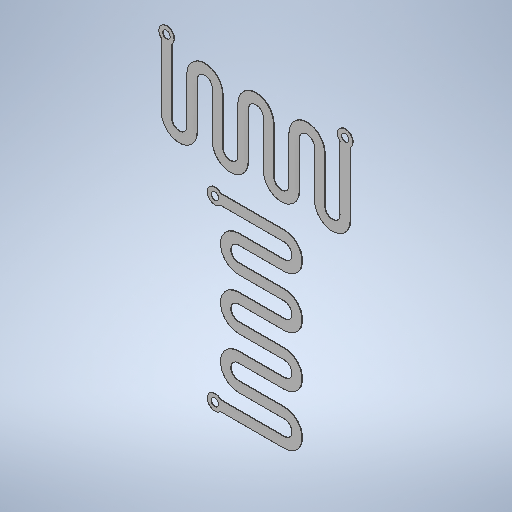
# Autodesk Inventor part: sensor_002_001
Saved by Autodesk Inventor 2025.2 (Build 292293000, 293)
## iProperties
Created: 2025-03-20
Part Number: sensor_002_001
Material: Genérico
Document SubType Name: Modeling
Designer: Carlos Dias
Density: 1 g/cm^3
Appearance: Padrão
Author: Carlos Dias
Autodesk Inventor part; units mm, degrees
ref_plane "YZ Plane" through (0, 0, 0) normal (1, 0, 0) x (0, 1, 0)
ref_plane "XZ Plane" through (0, 0, 0) normal (0, 1, 0) x (-1, 0, 0)
ref_plane "XY Plane" through (0, 0, 0) normal (0, 0, 1) x (1, 0, 0)
sketch "Esboço1" plane through (0, 0, 0) normal (0, 0, 1) x (1, 0, 0)
  circle A0 centre (-350, 253) radius 30 construction
  line L0 (0, 0) -> (0, 0) construction
  line L1 (0, 0) -> (0, 0) construction
  circle A1 centre (-350, 253) radius 15
  line L2 (-370, 230.6393) -> (-370, -19.3607)
  line L3 (-330, 230.6393) -> (-330, -19.3607)
  arc A2 (-330, 230.6393) -> (-370, 230.6393) centre (-350, 253) ccw
  circle A3 centre (-300, -19.3607) radius 30 construction
  line L4 (-270, 160.6393) -> (-270, -19.3607)
  line L5 (-230, 160.6393) -> (-230, -19.3607)
  circle A4 centre (-300, -19.3607) radius 70 construction
  arc A5 (-370, -19.3607) -> (-230, -19.3607) centre (-300, -19.3607) ccw
  arc A6 (-330, -19.3607) -> (-270, -19.3607) centre (-300, -19.3607) ccw
  line L6 (-330, 230.6393) -> (0, 230.6393) construction
  circle A7 centre (-200, 160.6393) radius 30 construction
  circle A8 centre (-200, 160.6393) radius 70 construction
  line L7 (-170, 160.6393) -> (-170, -19.3607)
  line L8 (-130, 160.6393) -> (-130, -19.3607)
  arc A9 (-170, 160.6393) -> (-230, 160.6393) centre (-200, 160.6393) ccw
  arc A10 (-130, 160.6393) -> (-270, 160.6393) centre (-200, 160.6393) ccw
  circle A11 centre (-100, -19.3607) radius 30 construction
  circle A12 centre (-100, -19.3607) radius 70 construction
  arc A13 (-130, -19.3607) -> (-70, -19.3607) centre (-100, -19.3607) ccw
  arc A14 (-170, -19.3607) -> (-30, -19.3607) centre (-100, -19.3607) ccw
  line L9 (-70, 160.6393) -> (-70, -19.3607)
  line L10 (-30, 160.6393) -> (-30, -19.3607)
  circle A15 centre (0, 160.6393) radius 30 construction
  circle A16 centre (0, 160.6393) radius 70 construction
  arc A17 (30, 160.6393) -> (-30, 160.6393) centre (0, 160.6393) ccw
  arc A18 (70, 160.6393) -> (-70, 160.6393) centre (0, 160.6393) ccw
  line L11 (70, 160.6393) -> (70, -19.3607)
  line L12 (30, 160.6393) -> (30, -19.3607)
  circle A19 centre (100, -19.3607) radius 30 construction
  circle A20 centre (100, -19.3607) radius 70 construction
  arc A21 (70, -19.3607) -> (130, -19.3607) centre (100, -19.3607) ccw
  arc A22 (30, -19.3607) -> (170, -19.3607) centre (100, -19.3607) ccw
  line L13 (130, 160.6393) -> (130, -19.3607)
  line L14 (170, 160.6393) -> (170, -19.3607)
  circle A23 centre (200, 160.6393) radius 30 construction
  circle A24 centre (200, 160.6393) radius 70 construction
  arc A25 (230, 160.6393) -> (170, 160.6393) centre (200, 160.6393) ccw
  arc A26 (270, 160.6393) -> (130, 160.6393) centre (200, 160.6393) ccw
  line L15 (230, 160.6393) -> (230, -19.3607)
  line L16 (270, 160.6393) -> (270, -19.3607)
  circle A27 centre (300, -19.3607) radius 30 construction
  circle A28 centre (300, -19.3607) radius 70 construction
  arc A29 (270, -19.3607) -> (330, -19.3607) centre (300, -19.3607) ccw
  arc A30 (230, -19.3607) -> (370, -19.3607) centre (300, -19.3607) ccw
  line L17 (330, 230.6393) -> (330, -19.3607)
  line L18 (370, 230.6393) -> (370, -19.3607)
  circle A31 centre (350, 253) radius 30 construction
  arc A32 (370, 230.6393) -> (330, 230.6393) centre (350, 253) ccw
  circle A33 centre (350, 253) radius 15
  line L19 (-350, 253) -> (350, 253) construction
  circle A34 centre (-160.6752, -200) radius 30 construction
  line L20 (0, 0) -> (-350, 0)
  circle A35 centre (-160.6752, -200) radius 15
  line L21 (-138.3146, -180) -> (111.6854, -180)
  line L22 (-138.3146, -220) -> (111.6854, -220)
  arc A36 (-138.3146, -180) -> (-138.3146, -220) centre (-160.6752, -200) ccw
  circle A37 centre (111.6854, -250) radius 30 construction
  circle A38 centre (111.6854, -250) radius 70 construction
  arc A39 (111.6854, -280) -> (111.6854, -220) centre (111.6854, -250) ccw
  arc A40 (111.6854, -320) -> (111.6854, -180) centre (111.6854, -250) ccw
  line L23 (-68.3146, -280) -> (111.6854, -280)
  line L24 (-68.3146, -320) -> (111.6854, -320)
  circle A41 centre (-68.3146, -350) radius 30 construction
  arc A42 (-68.3146, -320) -> (-68.3146, -380) centre (-68.3146, -350) ccw
  circle A43 centre (-68.3146, -350) radius 70 construction
  arc A44 (-68.3146, -280) -> (-68.3146, -420) centre (-68.3146, -350) ccw
  line L25 (-68.3146, -380) -> (111.6854, -380)
  line L26 (-68.3146, -420) -> (111.6854, -420)
  circle A45 centre (111.6854, -450) radius 30 construction
  circle A46 centre (111.6854, -450) radius 70 construction
  arc A47 (111.6854, -480) -> (111.6854, -420) centre (111.6854, -450) ccw
  arc A48 (111.6854, -520) -> (111.6854, -380) centre (111.6854, -450) ccw
  line L27 (-68.3146, -480) -> (111.6854, -480)
  line L28 (-68.3146, -520) -> (111.6854, -520)
  circle A49 centre (-68.3146, -550) radius 30 construction
  circle A50 centre (-68.3146, -550) radius 70 construction
  arc A51 (-68.3146, -520) -> (-68.3146, -580) centre (-68.3146, -550) ccw
  arc A52 (-68.3146, -480) -> (-68.3146, -620) centre (-68.3146, -550) ccw
  line L29 (-68.3146, -580) -> (111.6854, -580)
  line L30 (-68.3146, -620) -> (111.6854, -620)
  circle A53 centre (111.6854, -650) radius 30 construction
  circle A54 centre (111.6854, -650) radius 70 construction
  arc A55 (111.6854, -680) -> (108.1175, -620.2129) centre (111.6854, -650) ccw
  arc A56 (111.6854, -720) -> (111.6854, -580) centre (111.6854, -650) ccw
  line L31 (-68.3146, -720) -> (111.6854, -720)
  line L32 (-68.3146, -680) -> (111.6854, -680)
  circle A57 centre (-68.3146, -750) radius 30 construction
  circle A58 centre (-68.3146, -750) radius 70 construction
  arc A59 (-68.3146, -720) -> (-68.3146, -780) centre (-68.3146, -750) ccw
  arc A60 (-68.3146, -680) -> (-68.3146, -820) centre (-68.3146, -750) ccw
  line L33 (-68.3146, -780) -> (111.6854, -780)
  line L34 (-68.3146, -820) -> (111.6854, -820)
  circle A61 centre (111.6854, -850) radius 30 construction
  circle A62 centre (111.6854, -850) radius 70 construction
  arc A63 (111.6854, -880) -> (105.8073, -820.5815) centre (111.6854, -850) ccw
  arc A64 (111.6854, -920) -> (111.6854, -780) centre (111.6854, -850) ccw
  line L35 (-138.3146, -880) -> (111.6854, -880)
  line L36 (-138.3146, -920) -> (111.6854, -920)
  circle A65 centre (-160.6752, -900) radius 30 construction
  arc A66 (-138.3146, -880) -> (-138.3146, -920) centre (-160.6752, -900) ccw
  circle A67 centre (-160.6752, -900) radius 15
  line L37 (-160.6752, -200) -> (160.6752, -200) construction
  point P0 (-370, 105.6393)
  point P1 (0, 253)
  point P2 (-13.3146, -220)
  point P3 (-13.3146, -180)
  point P4 (0, -200)
  point P5 (-130, -19.3607)
  dimension "d0" = 253
  dimension "d2" = 60
  dimension "d3" = 30
  dimension "d5" = 40
  dimension "d6" = 250
  dimension "d7" = 60
  dimension "d8" = 40
  dimension "d13" = 40
  dimension "d14" = 200
  constraints: 76 end point, 73 point on circle, 58 centre point, 48 coincident, 36 horizontal alignment, 35 vertical alignment, 27 horizontal, 19 tangent, 17 vertical, 16 equal radius, 10 equal length, 5 midpoint, 3 concentric, 2 perpendicular, 1 parallel, 29 other
  measures "d0" distance from line of L0 A1.centre
  measures "d2" diameter of A0
  measures "d3" diameter of A1
  measures "d5" distance between parallel lines of L3 L2
  measures "d6" distance of L2.start L2.end
  measures "d7" diameter of A3
  measures "d8" distance between parallel lines of L4 L5
  measures "d13" distance of point (-13.315, -220) point (-13.315, -180)
  measures "d14" distance from line of L20 A34.centre
extrude "Extrusão1" add sketch "Esboço1" along normal blind 2 contours A2 L3 A6 L4 L20 L5 A5 L2 | L20 L4 A10 L8 L7 A9 L5 | L20 L8 A13 L9 L10 A14 L7 | L9 A18 L11 A21 L13 A26 L16 A29 L17 A32 L18 A30 L15 A25 L14 A22 L12 A17 L10 L20 | L21 A40 L24 A42 L25 A48 L28 A51 L29 A56 L31 A59 L33 A64 L36 A66 L35 A63 L34 A60 L32 A55 L30 A52 L27 A47 L26 A44 L23 A39 L22 A36
